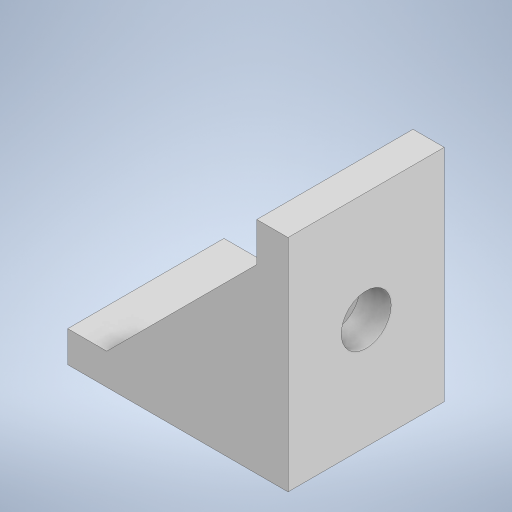
# Autodesk Inventor part: Escuadra DC
Saved by Autodesk Inventor 2024.2 (Build 282272000, 272)
## iProperties
Created: 2025-11-05
Part Number: Escuadra DC
Material: Generic
Document SubType Name: Modeling
Designer: ja.restrepo1
Density: 1 g/cm^3
Appearance: Default
Author: ja.restrepo1
Autodesk Inventor part; units mm, degrees
ref_plane "YZ Plane" through (0, 0, 0) normal (1, 0, 0) x (0, 1, 0)
ref_plane "XZ Plane" through (0, 0, 0) normal (0, 1, 0) x (-1, 0, 0)
ref_plane "XY Plane" through (0, 0, 0) normal (0, 0, 1) x (1, 0, 0)
sketch "Sketch1" plane through (0, 0, 0) normal (0, 0, 1) x (1, 0, 0)
  line L0 (14.1, 28.2) -> (14.1, 0)
  line L1 (14.1, 0) -> (-14.1, 0)
  line L2 (-14.1, 0) -> (-14.1, 4)
  line L3 (-14.1, 4) -> (10.1, 4)
  line L4 (10.1, 4) -> (10.1, 28.2)
  line L5 (10.1, 28.2) -> (14.1, 28.2)
  point P0 (0, 0)
  point P1 (0, 0)
  dimension "d0" = 28.2
  dimension "d1" = 4
  constraints: 12 end point, 7 perpendicular, 2 coincident, 1 midpoint, 1 vertical
  measures "d0" distance of L0.start L0.end
  measures "d1" distance of L1.end L2.end
extrude "Escuadra cuerpo" add sketch "Sketch1" along normal mid plane 20
sketch "Sketch2" plane through (0, 0, 10) normal (0, 0, 1) x (1, 0, 0)
  line L0 (10.1, 4) -> (-14.1, 4) projected
  line L1 (-9.1, 4) -> (10.1, 23.2)
  line L2 (10.1, 23.2) -> (10.1, 4)
  line L3 (10.1, 4) -> (-9.1, 4)
  line L4 (14.1, 28.2) -> (10.1, 28.2) projected
  point P0 (0, 0)
  dimension "d4" = 5
  dimension "d5" = 5
  constraints: 6 end point, 1 collinear, 1 perpendicular, 1 point on line
  measures "d4" distance of L0.end L1.start
  measures "d5" distance from line of L4 L1.end
extrude "Nervia lateral 1" add sketch "Sketch2" against normal blind 2.5
sketch "Sketch3" plane through (0, 0, -10) normal (0, 0, -1) x (-1, 0, 0)
  line L0 (-10.1, 4) -> (-10.1, 23.2) projected
  line L1 (-10.1, 23.2) -> (9.1, 4)
  line L2 (14.1, 4) -> (-10.1, 4) projected
  line L3 (-10.1, 4) -> (-10.1, 28.2) projected
  line L4 (-10.1, 23.2) -> (-10.1, 4)
  line L5 (-10.1, 4) -> (9.1, 4)
  point P0 (0, 0)
  dimension "d8" = 5
  dimension "d9" = 5
  constraints: 6 end point, 3 point on line, 1 collinear
  measures "d8" distance of L2.start L1.end
  measures "d9" distance of L3.end L0.end
extrude "Nervio lateral 2" add sketch "Sketch3" against normal blind 2.5
sketch "Sketch4" plane through (-14.1, 0, 10) normal (0, -1, 0) x (1, 0, 0)
  point P0 (14.1, -10)
  point P1 (14.1, -10)
  constraints: 1 coincident
hole "BCC M6 1" at (0, 0, 0) direction (0, 1, 0) diameter 6.4 end through all
sketch "Sketch5" plane through (14.1, 0, 10) normal (1, 0, 0) x (0, 0, -1)
  line L0 (0, 0) -> (0, 28.2) projected
  line L1 (20, 0) -> (0, 0) projected
  point P0 (10, 0)
  point P1 (10, 14.1)
  point P2 (0, 14.1)
  point P3 (10, 0)
  constraints: 2 midpoint, 1 horizontal alignment, 1 vertical alignment
hole "BCC M5 2" at (14.1, 14.1, 0) direction (-1, 0, 0) diameter 6.4 end through all
body "Solid1"
